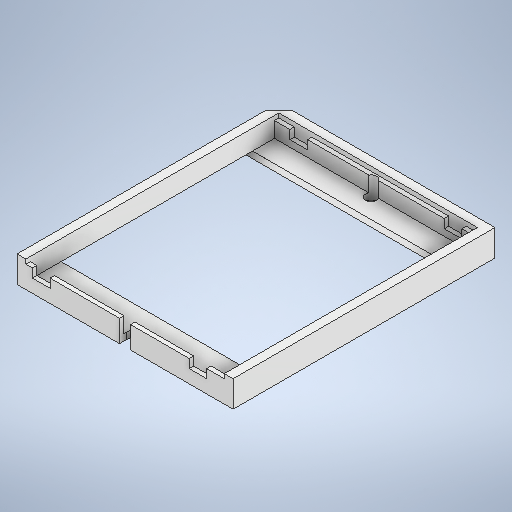
# Autodesk Inventor part: Digital Module Cover Reversed V3
Saved by Autodesk Inventor 2025 (Build 290162000, 162)
## iProperties
Created: 2023-10-04
Part Number: Digital Module Cover Reversed V3
Material: ABS Plastic
Document SubType Name: Modeling
Designer: cfang
Density: 1.06 g/cm^3
Appearance: Smooth - White
Author: cfang
Autodesk Inventor part; units mm, degrees
ref_plane "YZ Plane" through (0, 0, 0) normal (1, 0, 0) x (0, 1, 0)
ref_plane "XZ Plane" through (0, 0, 0) normal (0, 1, 0) x (-1, 0, 0)
ref_plane "XY Plane" through (0, 0, 0) normal (0, 0, 1) x (1, 0, 0)
sketch "Sketch1" plane through (0, 0, 0) normal (0, 1, 0) x (-1, 0, 0)
  line L0 (-24.55, -31.25) -> (24.55, -31.25)
  line L1 (24.55, -31.25) -> (24.55, 31.25)
  line L2 (24.55, 31.25) -> (-24.55, 31.25)
  line L3 (-24.55, 31.25) -> (-24.55, -31.25)
  line L4 (-24.55, -31.25) -> (24.55, 31.25) construction
  line L5 (24.55, -31.25) -> (-24.55, 31.25) construction
  point P0 (0, 0)
  dimension "d0" = 62.5
  dimension "d1" = 49.1
  constraints: 12 end point, 2 midpoint, 2 parallel, 1 horizontal, 1 perpendicular
  measures "d0" distance of L0.end L1.end
  measures "d1" distance of L1.end L2.end
extrude "Extrusion1" add sketch "Sketch1" along normal blind 6
sketch "Sketch2" plane through (0, 6, 0) normal (0, 1, 0) x (1, 0, 0)
  line L0 (22.55, 29.25) -> (-22.55, 29.25)
  line L1 (-22.55, 29.25) -> (-22.55, -29.25)
  line L2 (-22.55, -29.25) -> (22.55, -29.25)
  line L3 (22.55, -29.25) -> (22.55, 29.25)
  line L4 (22.55, 29.25) -> (-22.55, -29.25) construction
  line L5 (-22.55, 29.25) -> (22.55, -29.25) construction
  line L6 (-24.55, 31.25) -> (-24.55, -31.25) projected
  line L7 (-24.55, -31.25) -> (24.55, -31.25) projected
  point P0 (0, 0)
  dimension "d4" = 2
  dimension "d5" = 2
  constraints: 12 end point, 2 midpoint, 2 parallel, 1 horizontal, 1 perpendicular
  measures "d4" distance between parallel lines of L6 L1
  measures "d5" distance between parallel lines of L7 L2
extrude "Extrusion2" cut sketch "Sketch2" against normal blind 1
sketch "Sketch3" plane through (0, 5, 0) normal (0, 1, 0) x (1, 0, 0)
  line L0 (22.55, 28.25) -> (-22.55, 28.25)
  line L1 (-22.55, 28.25) -> (-22.55, -28.25)
  line L2 (-22.55, -28.25) -> (22.55, -28.25)
  line L3 (22.55, -28.25) -> (22.55, 28.25)
  line L4 (22.55, 28.25) -> (-22.55, -28.25) construction
  line L5 (-22.55, 28.25) -> (22.55, -28.25) construction
  line L6 (-22.55, 29.25) -> (22.55, 29.25) projected
  line L7 (-22.55, -29.25) -> (-22.55, 29.25) projected
  point P0 (0, 0)
  dimension "d48" = 1
  constraints: 12 end point, 2 midpoint, 2 parallel, 1 horizontal, 1 perpendicular, 1 point on line
  measures "d48" distance between parallel lines of L6 L0
extrude "Extrusion3" cut sketch "Sketch3" against normal blind 3.5
sketch "Sketch9" plane through (0, 6, 0) normal (0, 1, 0) x (1, 0, 0)
  line L0 (24.55, -28.25) -> (-24.55, -28.25)
  line L1 (-24.55, -28.25) -> (-24.55, -31.25)
  line L2 (-24.55, -31.25) -> (24.55, -31.25)
  line L3 (24.55, -31.25) -> (24.55, -28.25)
  line L4 (24.55, -31.25) -> (24.55, 31.25) projected
  line L5 (-22.55, 29.25) -> (22.55, 29.25) projected
  point P0 (0, 0)
  point P1 (-21.55, 29.25)
  point P2 (21.55, 29.25)
  dimension "d36" = 57.5
  constraints: 8 end point, 2 parallel, 1 horizontal, 1 perpendicular, 1 point on line
  measures "d36" distance between parallel lines of L0 L5
extrude "Extrusion7" cut sketch "Sketch9" against normal through all
sketch "Sketch10" plane through (0, 1.5, 0) normal (0, 1, 0) x (1, 0, 0)
  line L0 (22.55, -28.25) -> (-22.55, -28.25) projected
  line L1 (-22.55, -28.25) -> (22.55, -28.25)
  line L2 (22.55, -28.25) -> (22.55, -27.25)
  line L3 (22.55, -27.25) -> (-22.55, -27.25)
  line L4 (-22.55, -27.25) -> (-22.55, -28.25)
  point P0 (0, 0)
  point P1 (22.55, -28.25)
  dimension "d39" = 1
  constraints: 8 end point, 2 parallel, 1 horizontal, 1 perpendicular
  measures "d39" distance between parallel lines of L0 L3
extrude "Extrusion8" add sketch "Sketch10" along normal up to surface (3.5 mm away)
sketch "Sketch11" plane through (0, 1.5, 0) normal (0, 1, 0) x (1, 0, 0)
  circle A0 centre (0, 27.65) radius 1.25
  circle A1 centre (0, -26.65) radius 1.25
  line L0 (1.25, -26.65) -> (1.25, -28.25)
  line L1 (-22.55, -28.25) -> (22.55, -28.25) projected
  line L2 (-1.25, -26.65) -> (-1.25, -28.25)
  point P0 (0, 0)
  dimension "d42" = 2.5
  dimension "d43" = 2.5
  dimension "d44" = 54.3
  dimension "d45" = 27.65
  constraints: 4 end point, 2 centre point, 2 point on circle, 2 point on line, 2 vertical alignment, 1 parallel, 1 tangent, 1 vertical
  measures "d42" diameter of A0
  measures "d43" diameter of A1
  measures "d44" distance of A1.centre A0.centre
  measures "d45" distance of A0.centre point (0, 0)
extrude "Extrusion9" cut sketch "Sketch11" along normal through all both and the other way through all
sketch "Sketch12" plane through (0, 6, 0) normal (0, 1, 0) x (1, 0, 0)
  line L0 (24.55, 31.25) -> (-24.55, 31.25) projected
  line L1 (-21.55, 31.25) -> (-24.55, 28.25)
  line L2 (-24.55, 31.25) -> (-24.55, -28.25) projected
  point P0 (0, 0)
  dimension "d49" = 3
  dimension "d50" = 3
  constraints: 2 end point, 2 point on line
  measures "d49" distance of L0.end L1.end
  measures "d50" distance of L1.start L0.end
extrude "Extrusion10" cut sketch "Sketch12" against normal blind 10
sketch "Sketch13" plane through (-22.55, 5, 28.25) normal (0, 1, 0) x (1, 0, 0)
  line L0 (21.3, 0) -> (-2, 0) projected
  line L1 (0, 1) -> (21.3, 1) projected
  line L2 (1.5, 0) -> (5.5, 0)
  line L3 (5.5, 0) -> (5.5, 1)
  line L4 (5.5, 1) -> (1.5, 1)
  line L5 (1.5, 1) -> (1.5, 0)
  line L6 (37.1, 0) -> (41.1, 0)
  line L7 (41.1, 0) -> (41.1, 1)
  line L8 (41.1, 1) -> (37.1, 1)
  line L9 (37.1, 1) -> (37.1, 0)
  line L10 (0, 0) -> (0, 57.5) projected
  line L11 (45.1, 57.5) -> (45.1, 0) projected
  line L12 (0, 56.5) -> (21.4534, 56.5) projected
  line L13 (0, 57.5) -> (45.1, 57.5) projected
  line L14 (3.5, 56.5) -> (7.5, 56.5)
  line L15 (7.5, 56.5) -> (7.5, 57.5)
  line L16 (7.5, 57.5) -> (3.5, 57.5)
  line L17 (3.5, 57.5) -> (3.5, 56.5)
  line L18 (38.6, 56.5) -> (42.6, 56.5)
  line L19 (42.6, 56.5) -> (42.6, 57.5)
  line L20 (42.6, 57.5) -> (38.6, 57.5)
  line L21 (38.6, 57.5) -> (38.6, 56.5)
  point P0 (22.55, 28.25)
  point P1 (38.6, 57)
  point P2 (3.5, 57.5)
  point P3 (7.5, 56.5)
  point P4 (38.6, 57.5)
  point P5 (1.5, 1)
  point P6 (5.5, 0)
  dimension "d53" = 4
  dimension "d54" = 4
  dimension "d55" = 1.5
  dimension "d56" = 4
  dimension "d57" = 3.5
  dimension "d58" = 2.5
  dimension "d59" = 4
  dimension "d60" = 4
  constraints: 32 end point, 8 parallel, 8 point on line, 4 horizontal, 4 perpendicular, 1 midpoint
  measures "d53" distance between parallel lines of L5 L3
  measures "d54" distance between parallel lines of L9 L7
  measures "d55" distance between parallel lines of L10 L5
  measures "d56" distance between parallel lines of L7 L11
  measures "d57" distance between parallel lines of L17 L10
  measures "d58" distance between parallel lines of L19 L11
  measures "d59" distance from line of point (38.6, 57) L19
  measures "d60" distance between parallel lines of L17 L15
extrude "Extrusion11" cut sketch "Sketch13" against normal blind 2 contours L13 L19 L18 L21 | L0 L5 L1 L3 | L17 L13 L15 L12 | L9 L8 L7 L6
sketch "Sketch17" plane through (-24.55, 0, 28.25) normal (-1, 0, 0) x (0, 0, 1)
  line L0 (-56.5, 0) -> (0, 0) projected
  line L1 (-1, 1.5) -> (-56.5, 1.5) projected
  line L2 (-8, 0) -> (-51.5, 0)
  line L3 (-51.5, 0) -> (-51.5, 1.5)
  line L4 (-51.5, 1.5) -> (-8, 1.5)
  line L5 (-8, 1.5) -> (-8, 0)
  line L6 (0, 0) -> (0, 6) projected
  line L7 (-8, 1.5) -> (-6, 1.5)
  line L8 (-8, 0.5) -> (-8, 1.5)
  line L9 (-8, 0) -> (-7.25, 0.75)
  line L10 (-8, 0) -> (-6.9393, 0) construction
  line L11 (-7.25, 0.75) -> (-8, 1.5)
  line L12 (-51.5, 0) -> (-52.25, 0.75)
  line L13 (-51.5, 0) -> (-50.4393, 0) construction
  line L14 (-52.25, 0.75) -> (-51.5, 1.5)
  line L15 (-59.5, 0) -> (-59.5, 6) projected
  line L16 (-8, 0) -> (-51.5, 0)
  line L17 (-51.5, 1.5) -> (-8, 1.5)
  point P0 (-28.25, 0)
  dimension "d69" = 8
  dimension "d72" = 45
  dimension "d73" = 45
  dimension "d75" = 45
  dimension "d76" = 45
  dimension "d77" = 8
  constraints: 28 end point, 5 equal length, 4 horizontal, 2 perpendicular, 2 point on line
  measures "d69" distance between parallel lines of L6 L5
  measures "d72" angle of L10 L9
  measures "d73" angle of L1 L11
  measures "d75" angle of L3 L12
  measures "d76" angle of L14 L3
  measures "d77" distance between parallel lines of L15 L3
extrude "Extrusion13" cut sketch "Sketch17" against normal through all
extrude "Extrusion14" [suppressed]
sketch "Sketch18" plane through (24.55, 0, -31.25) normal (1, 0, 0) x (0, 0, -1)
  line L0 (-7.25, 0.75) -> (-8, 0) projected
  line L1 (-51.5, 0) -> (-59.5, 0) projected
  line L2 (-8, 0) -> (-51.5, 0)
  line L3 (-8, 1.5) -> (-7.25, 0.75) projected
  line L4 (-51.5, 1.5) -> (-8, 1.5) projected
  line L5 (-52.25, 0.75) -> (-51.5, 1.5) projected
  line L6 (-51.5, 0) -> (-52.25, 0.75) projected
  point P0 (-31.25, 0)
  constraints: 2 end point, 1 horizontal
extrude "Extrusion15" add sketch "Sketch18" against normal blind 4.1
equation "\"d5\" = d4"
equation "\"d43\" = d42"
equation "\"d50\" = d49"
equation "\"d73\" = d72"
equation "\"d76\" = d75"
body "Solid1"
